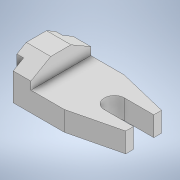
# Autodesk Inventor part: FINGER GUIDE
Saved by Autodesk Inventor 2022.4 (Build 264492000, 492)
## iProperties
Created: 2024-01-25
Part Number: FINGER GUIDE
Material: Generic
Document SubType Name: Modeling
Designer: t60147996
Density: 1 g/cm^3
Appearance: Default
Author: t60147996
Autodesk Inventor part; units mm, degrees
ref_plane "YZ Plane" through (0, 0, 0) normal (1, 0, 0) x (0, 1, 0)
ref_plane "XZ Plane" through (0, 0, 0) normal (0, 1, 0) x (-1, 0, 0)
ref_plane "XY Plane" through (0, 0, 0) normal (0, 0, 1) x (1, 0, 0)
sketch "Sketch1" plane through (0, 0, 0) normal (0, 1, 0) x (-1, 0, 0)
  line L0 (-52.324, -29.21) -> (52.324, -29.21)
  line L1 (52.324, -29.21) -> (52.324, 29.21)
  line L2 (52.324, 29.21) -> (-52.324, 29.21)
  line L3 (-52.324, 29.21) -> (-52.324, -29.21)
  line L4 (-52.324, -29.21) -> (52.324, 29.21) construction
  line L5 (52.324, -29.21) -> (-52.324, 29.21) construction
  point P0 (0, 0)
  dimension "d0" = 104.648
  dimension "d1" = 58.42
  constraints: 12 end point, 2 midpoint, 2 parallel, 1 horizontal, 1 perpendicular
  measures "d0" distance of L2.end L1.end
  measures "d1" distance of L1.end L0.end
extrude "Extrusion1" add sketch "Sketch1" along normal blind 38.1
sketch "Sketch2" plane through (-52.324, 0, 29.21) normal (0, 0, 1) x (1, 0, 0)
  line L0 (0, 38.1) -> (104.648, 38.1) projected
  line L1 (104.648, 0) -> (104.648, 38.1) projected
  line L2 (23.876, 38.1) -> (104.648, 38.1)
  line L3 (104.648, 38.1) -> (104.648, 19.304)
  line L4 (104.648, 19.304) -> (23.876, 19.304)
  line L5 (23.876, 19.304) -> (23.876, 38.1)
  line L6 (0, 0) -> (0, 38.1) projected
  line L7 (0, 0) -> (104.648, 0) projected
  point P0 (52.324, 0)
  dimension "d4" = 23.876
  dimension "d5" = 19.304
  constraints: 8 end point, 2 parallel, 2 point on line, 1 horizontal, 1 perpendicular
  measures "d4" distance between parallel lines of L5 L6
  measures "d5" distance between parallel lines of L4 L7
extrude "Extrusion2" cut sketch "Sketch2" against normal through all contours L0 L1 L4 L5
sketch "Sketch3" plane through (-52.324, 0, -29.21) normal (-1, 0, 0) x (0, 0, 1)
  line L0 (0, 38.1) -> (58.42, 38.1) projected
  line L1 (39.0626, 38.1) -> (58.42, 26.924)
  line L2 (58.42, 0) -> (58.42, 38.1) projected
  point P0 (29.21, 0)
  dimension "d8" = 11.176
  dimension "d9" = 30
  constraints: 2 end point, 2 point on line
  measures "d8" distance from line of L1.end L0
  measures "d9" angle of L1 L0
extrude "Extrusion3" cut sketch "Sketch3" against normal through all
sketch "Sketch4" plane through (-52.324, 0, -29.21) normal (-1, 0, 0) x (0, 0, 1)
  line L0 (0, 38.1) -> (39.0626, 38.1) projected
  line L1 (19.3574, 38.1) -> (0, 26.924)
  line L2 (0, 38.1) -> (0, 19.304) projected
  point P0 (29.21, 0)
  dimension "d12" = 11.176
  dimension "d13" = 30
  constraints: 2 end point, 2 point on line
  measures "d12" distance from line of L1.end L0
  measures "d13" angle of L1 L0
extrude "Extrusion4" cut sketch "Sketch4" against normal through all
sketch "Sketch5" plane through (-28.448, 19.304, 29.21) normal (0, 1, 0) x (1, 0, 0)
  line L0 (80.772, 0) -> (0, 0) projected
  line L1 (32.512, 0) -> (80.772, 11.684)
  line L2 (80.772, 58.42) -> (80.772, 0) projected
  point P0 (28.448, 29.21)
  dimension "d16" = 48.26
  dimension "d17" = 11.684
  constraints: 2 end point, 2 point on line
  measures "d16" distance from line of L1.start L2
  measures "d17" distance from line of L1.end L0
extrude "Extrusion5" cut sketch "Sketch5" against normal through all
sketch "Sketch6" plane through (-28.448, 19.304, -29.21) normal (0, 1, 0) x (1, 0, 0)
  line L0 (80.772, 0) -> (-23.876, 0) projected
  line L1 (32.512, 0) -> (80.772, -11.684)
  line L2 (80.772, 0) -> (80.772, -46.736) projected
  point P0 (28.448, -29.21)
  dimension "d20" = 11.684
  dimension "d21" = 48.26
  constraints: 2 end point, 2 point on line
  measures "d20" distance from line of L1.end L0
  measures "d21" distance from line of L1.start L2
extrude "Extrusion6" cut sketch "Sketch6" against normal through all
sketch "Sketch7" plane through (0, 0, 0) normal (0, -1, 0) x (1, 0, 0)
  line L0 (-52.324, 29.21) -> (-52.324, 9.8526) projected
  line L1 (-52.324, 19.5313) -> (-45.72, 19.5313)
  line L2 (-45.72, 19.5313) -> (-45.72, 29.6913)
  line L3 (-45.72, 29.6913) -> (-52.324, 29.6913)
  line L4 (-52.324, 29.6913) -> (-52.324, 19.5313)
  point P0 (0, 0)
  dimension "d25" = 6.604
  dimension "d26" = 10.16
  constraints: 8 end point, 2 parallel, 1 horizontal, 1 midpoint, 1 perpendicular
  measures "d25" distance of L3.end L2.end
  measures "d26" distance of L2.end L1.end
extrude "Extrusion7" cut sketch "Sketch7" against normal through all
sketch "Sketch8" plane through (0, 0, 0) normal (0, -1, 0) x (1, 0, 0)
  line L0 (-52.324, -9.8526) -> (-52.324, -29.21) projected
  line L1 (-52.324, -19.5313) -> (-45.72, -19.5313)
  line L2 (-45.72, -19.5313) -> (-45.72, -29.6913)
  line L3 (-45.72, -29.6913) -> (-52.324, -29.6913)
  line L4 (-52.324, -29.6913) -> (-52.324, -19.5313)
  point P0 (0, 0)
  dimension "d29" = 6.604
  dimension "d30" = 10.16
  constraints: 8 end point, 2 parallel, 1 horizontal, 1 midpoint, 1 perpendicular
  measures "d29" distance of L2.end L3.end
  measures "d30" distance of L1.end L2.end
extrude "Extrusion8" cut sketch "Sketch8" against normal through all
sketch "Sketch9" plane through (-28.448, 19.304, 29.21) normal (0, 1, 0) x (1, 0, 0)
  line L0 (80.772, 46.736) -> (80.772, 11.684) projected
  circle A0 centre (52.324, 29.21) radius 9.906
  point P0 (28.448, 29.21)
  point P1 (80.772, 29.21)
  point P2 (80.772, 29.21)
  dimension "d35" = 19.812
  dimension "d36" = 28.448
  constraints: 2 horizontal alignment, 2 midpoint, 1 centre point
  measures "d35" diameter of A0
  measures "d36" distance from line of L0 A0.centre
extrude "Extrusion9" cut sketch "Sketch9" against normal through all
sketch "Sketch10" plane through (-28.448, 19.304, 29.21) normal (0, 1, 0) x (1, 0, 0)
  circle A0 centre (52.324, 29.21) radius 9.906 projected
  line L0 (80.772, 11.684) -> (80.772, 46.736) projected
  line L1 (52.324, 39.116) -> (80.772, 39.116)
  line L2 (80.772, 39.116) -> (80.772, 19.304)
  line L3 (80.772, 19.304) -> (52.324, 19.304)
  line L4 (52.324, 19.304) -> (52.324, 39.116)
  point P0 (28.448, 29.21)
  dimension "d39" = 19.812
  constraints: 8 end point, 2 parallel, 1 horizontal, 1 perpendicular, 1 point on line, 2 other
  measures "d39" distance of L1.end L2.end
extrude "Extrusion10" cut sketch "Sketch10" against normal through all contours A0 L1 L0 L3
sketch "Sketch11" plane through (0, 0, 0) normal (0, -1, 0) x (1, 0, 0)
  line L0 (-52.324, -19.5313) -> (-52.324, 19.5313) projected
  line L1 (-52.324, -19.5313) -> (-45.72, -19.5313)
  line L2 (-45.72, -19.5313) -> (-45.72, -19.0233)
  line L3 (-45.72, -19.0233) -> (-52.324, -19.0233)
  line L4 (-52.324, -19.0233) -> (-52.324, -19.5313)
  point P0 (0, 0)
  dimension "d42" = 0.508
  constraints: 8 end point, 2 parallel, 1 horizontal, 1 perpendicular
  measures "d42" distance of L2.end L1.end
sketch "Sketch12" plane through (0, 0, 0) normal (0, -1, 0) x (1, 0, 0)
  line L0 (-52.324, -19.5313) -> (-52.324, 19.5313) projected
  line L1 (-52.324, 19.5313) -> (-45.72, 19.5313)
  line L2 (-45.72, 19.5313) -> (-45.72, 19.0233)
  line L3 (-45.72, 19.0233) -> (-52.324, 19.0233)
  line L4 (-52.324, 19.0233) -> (-52.324, 19.5313)
  point P0 (0, 0)
  dimension "d43" = 0.508
  constraints: 8 end point, 2 parallel, 1 horizontal, 1 perpendicular
  measures "d43" distance of L1.end L2.end
extrude "Extrusion11" cut sketch "Sketch11" against normal through all
extrude "Extrusion12" cut sketch "Sketch12" against normal through all
body "Solid1"
